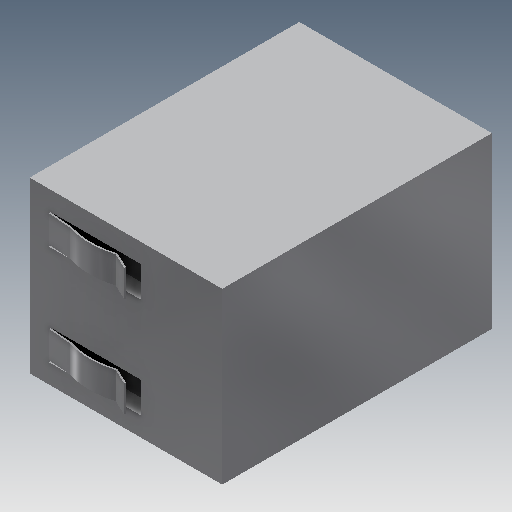
# Autodesk Inventor part: config - nic module
Saved by Autodesk Inventor 2019.1 (Build 231200000, 200)
## iProperties
Company: Autodesk Asia Pte. Ltd.
Created: 2005-11-27
Part Number: config - nic module
Document SubType Name: Modeling
Designer: Simon.Ng@autodesk.com
Stock Number: config - nic module
Density: 1 g/cm^3
Material: Generic
Mass: 13.2374 g
Surface Area: 91.9014 cm^2
Volume: 13.2374 cm^3
Appearance: Aluminum - Polished
Title: PC Demo
Author: Simon.Ng@autodesk.com
Autodesk Inventor part; units mm, degrees
ref_plane "YZ Plane" through (0, 0, 0) normal (1, 0, 0) x (0, 1, 0)
ref_plane "XZ Plane" through (0, 0, 0) normal (0, 1, 0) x (-1, 0, 0)
ref_plane "XY Plane" through (0, 0, 0) normal (0, 0, 1) x (1, 0, 0)
sketch "Sketch1" plane through (0, 0, 0) normal (0, 0, 1) x (1, 0, 0)
  line L0 (0, 17.6) -> (0, -13.2) projected
  line L1 (-2.5, 0) -> (32.5, 0) projected
  line L2 (0, 11) -> (25, 11)
  line L3 (25, 11) -> (25, -11)
  line L4 (25, -11) -> (0, -11)
  line L5 (0, -11) -> (0, 11)
  dimension "d0" = 22
  dimension "d1" = 25
  constraints: 8 end point, 2 parallel, 1 horizontal, 1 perpendicular, 1 point on line, 1 other
  measures "d0" distance of L2.end L3.end
  measures "d1" distance of L2.start L2.end
extrude "Extrusion1" add sketch "Sketch1" along normal blind 35
sketch "Sketch2" plane through (0, -11, 0) normal (-1, 0, 0) x (0, 0, 1)
  line L0 (0, 0) -> (0, 22) projected
  line L1 (-3.5, 11) -> (45.5, 11) projected
  line L2 (4, 18.5) -> (10, 18.5)
  line L3 (10, 18.5) -> (10, 3.5)
  line L4 (10, 3.5) -> (4, 3.5)
  line L5 (4, 3.5) -> (4, 18.5)
  line L6 (12.5, 18.5) -> (18.5, 18.5)
  line L7 (18.5, 18.5) -> (18.5, 3.5)
  line L8 (18.5, 3.5) -> (12.5, 3.5)
  line L9 (12.5, 3.5) -> (12.5, 18.5)
  line L10 (20.5, 18.5) -> (27.5, 18.5)
  line L11 (27.5, 18.5) -> (27.5, 3.5)
  line L12 (27.5, 3.5) -> (20.5, 3.5)
  line L13 (20.5, 3.5) -> (20.5, 18.5)
  line L14 (27.5, 17) -> (31.5, 17)
  line L15 (31.5, 17) -> (31.5, 5)
  line L16 (31.5, 5) -> (27.5, 5)
  line L17 (27.5, 5) -> (27.5, 17)
  dimension "d4" = 4
  dimension "d5" = 15
  dimension "d6" = 2.5
  dimension "d7" = 6
  dimension "d8" = 11
  dimension "d9" = 2
  dimension "d10" = 7
  dimension "d11" = 12
  constraints: 32 end point, 8 parallel, 5 collinear, 4 horizontal, 4 perpendicular, 1 point on line, 2 other
  measures "d4" distance between parallel lines of L0 L5
  measures "d5" distance of L4.end L2.start
  measures "d6" distance between parallel lines of L9 L3
  measures "d7" distance of L3.end L4.end
  measures "d8" distance between parallel lines of L15 L13
  measures "d9" distance between parallel lines of L7 L13
  measures "d10" distance of L10.start L10.end
  measures "d11" distance of L14.end L15.end
extrude "Extrusion2" cut sketch "Sketch2" against normal blind 20
sketch "Sketch3" plane through (20, -11, 0) normal (-1, 0, 0) x (0, 0, 1)
  line L0 (10, 3.5) -> (10, 18.5) projected
  line L1 (9, 18) -> (7.5, 18)
  line L2 (7.5, 18) -> (7.5, 4)
  line L3 (7.5, 4) -> (9, 4)
  line L4 (9, 4) -> (9, 18)
  line L5 (17.5, 18) -> (16, 18)
  line L6 (16, 18) -> (16, 4)
  line L7 (16, 4) -> (17.5, 4)
  line L8 (17.5, 4) -> (17.5, 18)
  line L9 (12.5, 18.5) -> (12.5, 3.5) projected
  line L10 (12.5, 3.5) -> (18.5, 3.5) projected
  line L11 (18.5, 3.5) -> (18.5, 18.5) projected
  line L12 (18.5, 18.5) -> (12.5, 18.5) projected
  line L13 (-3.5, 11) -> (45.5, 11) projected
  dimension "d14" = 1.5
  dimension "d15" = 1
  dimension "d16" = 1
  dimension "d17" = 14
  constraints: 16 end point, 4 parallel, 2 equal length, 2 horizontal, 2 perpendicular, 2 other
  measures "d14" distance of L1.start L1.end
  measures "d15" distance between parallel lines of L0 L4
  measures "d16" distance between parallel lines of L11 L8
  measures "d17" distance of L1.end L2.end
extrude "Extrusion3" add sketch "Sketch3" along normal blind 18 contours L4 L13 L2 L1 | L4 L3 L2 L13 | L8 L13 L6 L5 | L8 L7 L6 L13
sketch "Sketch4" plane through (0, 0, 0) normal (0, 1, 0) x (-1, 0, 0)
  line L0 (-20, 27.5) -> (-20, 20.5) projected
  line L1 (0, 20.5) -> (-20, 20.5) projected
  line L2 (-20, 23) -> (-2, 20.5)
  line L3 (0, 0) -> (0, 35) projected
  dimension "d20" = 2
  dimension "d21" = 2.5
  constraints: 2 coincident, 2 end point, 2 point on line
  measures "d20" distance from line of L3 point (-2, 20.5)
  measures "d21" distance from line of L1 L2.start
extrude "Extrusion4" add sketch "Sketch4" along normal mid plane 10
sketch "Sketch5" plane through (20, -11, 0) normal (-1, 0, 0) x (0, 0, 1)
  line L0 (20.5, 16) -> (23, 16) projected
  line L1 (23, 16) -> (23, 6) projected
  line L2 (20.5, 3.5) -> (20.5, 18.5) projected
  line L3 (20.5, 15.8) -> (23, 15.8)
  line L4 (23, 15.8) -> (23, 15.3)
  line L5 (23, 15.3) -> (20.5, 15.3)
  line L6 (20.5, 15.3) -> (20.5, 15.8)
  dimension "d24" = 0.2
  dimension "d25" = 0.5
  constraints: 8 end point, 2 parallel, 2 point on line, 1 horizontal, 1 perpendicular
  measures "d24" distance between parallel lines of L3 L0
  measures "d25" distance between parallel lines of L5 L3
extrude "Extrusion5" cut sketch "Sketch5" along normal through all contours L3 L1 L5 L2
pattern_linear "Rectangular Pattern1" count 14 spacing 0.7 along (0, -1, 0) of "Extrusion5"
sketch "Sketch6" plane through (0, 0, 35) normal (0, 0, 1) x (1, 0, 0)
  line L0 (0, 11) -> (25, 11) projected
  line L1 (0, -11) -> (0, 11) projected
  line L2 (2.5, 8.5) -> (14.5, 8.5)
  line L3 (14.5, 8.5) -> (14.5, 4.5)
  line L4 (14.5, 4.5) -> (2.5, 4.5)
  line L5 (2.5, 4.5) -> (2.5, 8.5)
  dimension "d31" = 2.5
  dimension "d32" = 12
  dimension "d33" = 4
  dimension "d34" = 2.5
  constraints: 8 end point, 2 parallel, 1 horizontal, 1 perpendicular
  measures "d31" distance between parallel lines of L0 L2
  measures "d32" distance of L2.start L2.end
  measures "d33" distance of L2.end L3.end
  measures "d34" distance between parallel lines of L1 L5
extrude "Extrusion6" cut sketch "Sketch6" against normal blind 2
ref_plane "Work Plane1" through (2.5, 6.5, 33) normal (0, -1, 0) x (1, 0, 0)
sketch "Sketch7" plane through (2.5, 6.5, 33) normal (0, -1, 0) x (1, 0, 0)
  line L0 (0, 2) -> (0, 0) construction
  line L1 (0, 2) -> (3.0475, 2.2666)
  line L2 (8.95, 2.2854) -> (11, 3.2413)
  arc A0 (8.95, 2.2854) -> (3.0475, 2.2666) centre (6.0291, -7.2785) ccw
  line L3 (0, 1.7992) -> (3.0866, 2.0693)
  arc A1 (8.9646, 2.0715) -> (3.0866, 2.0693) centre (6.0291, -7.2785) ccw
  line L4 (8.9646, 2.0715) -> (11.0845, 3.06)
  line L5 (11, 3.2413) -> (11.0845, 3.06)
  line L6 (0, 2) -> (0, 1.7992)
  dimension "d37" = 11
  dimension "d38" = 95
  dimension "d39" = 10
  dimension "d40" = 65
  dimension "d41" = 0.2
  constraints: 13 end point, 4 point on circle, 2 centre point, 1 perpendicular, 1 point on line, 1 other
  measures "d37" distance from line of L0 L2.end
  measures "d38" angle of L0 L1
  measures "d39" radius of A0
  measures "d40" angle of L0 L2
  measures "d41" distance between parallel lines of L3 L1
extrude "Extrusion7" add sketch "Sketch7" along normal mid plane 3.5
mirror "Mirror1" about plane through (0, 0, 0) normal (0, 1, 0) of "Extrusion6", "Extrusion7"
equation "\"d16\" = d15"
body "Solid1"
